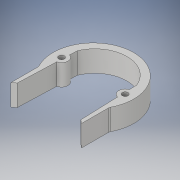
# Autodesk Inventor part: Motor Plate Cover
Saved by Autodesk Inventor 2019.2 (Build 232265000, 265)
## iProperties
Created: 2018-12-29
Part Number: Motor Plate Cover
Material: Generic
Document SubType Name: Modeling
Designer: Petar
Density: 1 g/cm^3
Appearance: Default
Author: Petar
Autodesk Inventor part; units mm, degrees
ref_plane "YZ Plane" through (0, 0, 0) normal (1, 0, 0) x (0, 1, 0)
ref_plane "XZ Plane" through (0, 0, 0) normal (0, 1, 0) x (-1, 0, 0)
ref_plane "XY Plane" through (0, 0, 0) normal (0, 0, 1) x (1, 0, 0)
derived "Motor Holder.ipt"
sketch "Sketch8" plane through (0, -4, 0) normal (0, -1, 0) x (1, 0, 0)
  arc A0 (-13.1442, -11.0271) -> (-17.3442, -11.0271) centre (-15.2442, -11.0271) ccw
  line L0 (-13.1442, -11.0271) -> (-13.1442, -17.0271)
  arc A1 (-17.3442, -17.0271) -> (-13.1442, -17.0271) centre (-15.2442, -17.0271) ccw
  line L1 (-17.3442, -17.0271) -> (-17.3442, -11.0271)
  arc A2 (17.3442, -11.0271) -> (13.1442, -11.0271) centre (15.2442, -11.0271) ccw
  line L2 (17.3442, -11.0271) -> (17.3442, -17.0271)
  arc A3 (13.1442, -17.0271) -> (17.3442, -17.0271) centre (15.2442, -17.0271) ccw
  line L3 (13.1442, -17.0271) -> (13.1442, -11.0271)
  arc A4 (13.1442, -47.5154) -> (17.3442, -47.5154) centre (15.2442, -47.5154) ccw
  line L4 (13.1442, -47.5154) -> (13.1442, -41.5154)
  arc A5 (17.3442, -41.5154) -> (13.1442, -41.5154) centre (15.2442, -41.5154) ccw
  line L5 (17.3442, -41.5154) -> (17.3442, -47.5154)
  arc A6 (-17.3442, -47.5154) -> (-13.1442, -47.5154) centre (-15.2442, -47.5154) ccw
  line L6 (-17.3442, -47.5154) -> (-17.3442, -41.5154)
  arc A7 (-13.1442, -41.5154) -> (-17.3442, -41.5154) centre (-15.2442, -41.5154) ccw
  line L7 (-13.1442, -41.5154) -> (-13.1442, -47.5154)
  line L8 (25, -14.8404) -> (25, 33.7287)
  arc A8 (25, 33.7287) -> (-25, 33.7287) centre (0, 33.7287) ccw
  line L9 (-25, 33.7287) -> (-25, -14.8404)
  arc A9 (-25.3333, -16.2148) -> (-25, -14.8404) centre (-28, -14.8404) ccw
  arc A10 (-25.3333, -16.2148) -> (25.3333, -16.2148) centre (0, -29.2713) ccw
  arc A11 (25, -14.8404) -> (25.3333, -16.2148) centre (28, -14.8404) ccw
  circle A12 centre (22.5, -29.2713) radius 2
  circle A13 centre (-22.5, -29.2713) radius 2
  arc A14 (-11, -34.3161) -> (11, -34.3161) centre (0, -34.3161) ccw
  line L10 (-11, -34.3161) -> (-11, -24.3161)
  arc A15 (11, -24.3161) -> (-11, -24.3161) centre (0, -24.3161) ccw
  line L11 (11, -24.3161) -> (11, -34.3161)
  circle A16 centre (0, 33.7287) radius 13.5
  point P0 (0, 0)
sketch "Sketch2" plane through (0, 0, 0) normal (0, 1, 0) x (-1, 0, 0)
  arc A0 (-25.3333, -16.2148) -> (25.3333, -16.2148) centre (0, -29.2713) ccw projected
  arc A1 (25, -14.8404) -> (25.3333, -16.2148) centre (28, -14.8404) ccw projected
  line L0 (25, 33.7287) -> (25, -14.8404) projected
  line L1 (-25, -14.8404) -> (-25, 33.7287) projected
  arc A2 (-25.3333, -16.2148) -> (-25, -14.8404) centre (-28, -14.8404) ccw projected
  circle A3 centre (22.5, -29.2713) radius 2 projected
  circle A4 centre (-22.5, -29.2713) radius 2 projected
  arc A5 (-11, -34.3161) -> (11, -34.3161) centre (0, -34.3161) ccw projected
  arc A6 (11, -24.3161) -> (-11, -24.3161) centre (0, -24.3161) ccw projected
  line L2 (11, -34.3161) -> (11, -24.3161) projected
  line L3 (-11, -24.3161) -> (-11, -34.3161) projected
  arc A7 (-25, 4) -> (25, 4) centre (0, 35.225) ccw
  line L4 (0, 0) -> (0, -57.7713) construction
  line L5 (22.5, 2.1531) -> (21.5146, -24.8805)
  arc A8 (21.5146, -24.8805) -> (21.1976, -33.5787) centre (22.5, -29.2713) ccw
  line L6 (21.1976, -33.5787) -> (21.0005, -38.9874)
  arc A9 (0, -53) -> (21.0005, -38.9874) centre (0, -30.2572) ccw
  arc A10 (-21.1976, -33.5787) -> (-21.5146, -24.8805) centre (-22.5, -29.2713) ccw
  line L7 (-21.1976, -33.5787) -> (-21.0005, -38.9874)
  arc A11 (-21.0005, -38.9874) -> (0, -53) centre (0, -30.2572) ccw
  line L8 (-22.5, 2.1531) -> (-21.5146, -24.8805)
  dimension "d1" = 40
  dimension "d5" = 2.5
  dimension "d6" = 2.5
  constraints: 13 point on circle, 10 end point, 6 symmetric about line, 5 centre point, 3 point on line, 1 coincident, 1 collinear, 1 line through centre, 2 other
  measures "d1" radius of A7
  measures "d5" radial gap between concentric circles of A3 A8
  measures "d6" distance from line of L0 L5.start
extrude "Extrusion1" add sketch "Sketch2" along normal blind 15 contours A2 L1 A7 L8 A10 L7 A11 A9 L6 A8 L5 L0 A1 A0
body "Solid1"
